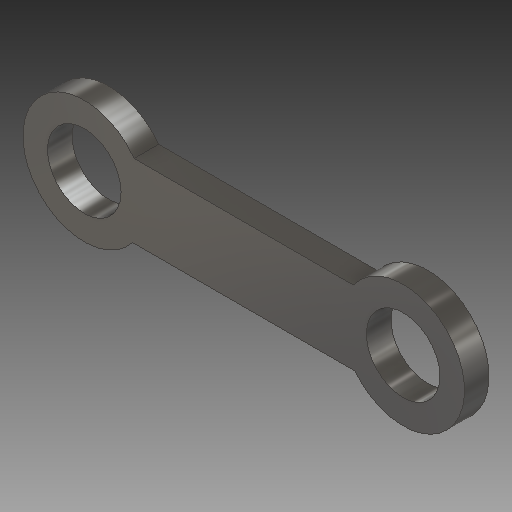
# Autodesk Inventor part: ConnectBar
Saved by Autodesk Inventor 2019 (Build 230136000, 136)
## iProperties
Created: 2018-12-28
Part Number: ConnectBar
Material: 钢，高强度，低合金
Document SubType Name: Modeling
Designer: JianQiao Hu
Density: 7.85 g/cm^3
Appearance: 钢 - 抛光
Author: JianQiao Hu
Autodesk Inventor part; units mm, degrees
ref_plane "YZ Plane" through (0, 0, 0) normal (1, 0, 0) x (0, 1, 0)
ref_plane "XZ Plane" through (0, 0, 0) normal (0, 1, 0) x (-1, 0, 0)
ref_plane "XY Plane" through (0, 0, 0) normal (0, 0, 1) x (1, 0, 0)
sketch "草图1" plane through (0, 0, 0) normal (0, 0, 1) x (1, 0, 0)
  circle A0 centre (-65, 0.3085) radius 15
  circle A1 centre (65, 0.3085) radius 15
  arc A2 (-44.698, 14.8971) -> (-45.3152, -15.1029) centre (-65, 0.3085) ccw
  arc A3 (45.3152, -15.1029) -> (44.698, 14.8971) centre (65, 0.3085) ccw
  line L0 (0, 0) -> (0, 60.3628)
  line L1 (0, 0) -> (-51.6716, 0)
  line L2 (-44.698, 14.8971) -> (44.698, 14.8971)
  line L3 (45.3152, -15.1029) -> (-45.3152, -15.1029)
  line L4 (-44.698, 14.8971) -> (45.3152, -15.1029) construction
  line L5 (44.698, 14.8971) -> (-45.3152, -15.1029) construction
  dimension "d0" = 30
  dimension "d1" = 30
  dimension "d2" = 50
  dimension "d3" = 50
  dimension "d4" = 65
  dimension "d6" = 65
  dimension "d9" = 30
  constraints: 12 end point, 4 centre point, 4 point on circle, 2 coincident, 2 horizontal, 2 point on line, 1 parallel, 1 vertical
  measures "d0" diameter of A0
  measures "d1" diameter of A1
  measures "d2" diameter of A2
  measures "d3" diameter of A3
  measures "d4" distance from line of L0 A0.centre
  measures "d6" distance from line of L0 A1.centre
  measures "d9" distance between parallel lines of L2 L3
extrude "拉伸1" add sketch "草图1" along normal blind 10
